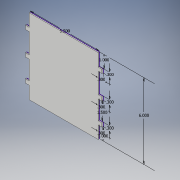
# Autodesk Inventor part: BB Gun Back Panel
Saved by Autodesk Inventor 2018 (Build 220112000, 112)
## iProperties
Created: 2019-05-24
Part Number: BB Gun Back Panel
Material: Generic
Document SubType Name: Modeling
Designer: 871357
Density: 1 g/cm^3
Appearance: Default
Author: 871357
Autodesk Inventor part; units mm, degrees
ref_plane "YZ Plane" through (0, 0, 0) normal (1, 0, 0) x (0, 1, 0)
ref_plane "XZ Plane" through (0, 0, 0) normal (0, 1, 0) x (-1, 0, 0)
ref_plane "XY Plane" through (0, 0, 0) normal (0, 0, 1) x (1, 0, 0)
sketch "Sketch1" plane through (0, 0, 0) normal (0, 0, 1) x (1, 0, 0)
  line L0 (0, 0) -> (139.7, 0)
  line L1 (139.7, 0) -> (139.7, 152.4)
  line L2 (139.7, 152.4) -> (0, 152.4)
  line L3 (139.7, 127) -> (147.32, 127)
  line L4 (147.32, 127) -> (147.32, 119.38)
  line L5 (147.32, 119.38) -> (139.7, 119.38)
  line L6 (139.7, 119.38) -> (139.7, 127)
  line L7 (139.7, 78.74) -> (147.32, 78.74)
  line L8 (147.32, 78.74) -> (147.32, 71.12)
  line L9 (147.32, 71.12) -> (139.7, 71.12)
  line L10 (139.7, 71.12) -> (139.7, 78.74)
  line L11 (139.7, 33.02) -> (147.32, 33.02)
  line L12 (147.32, 33.02) -> (147.32, 25.4)
  line L13 (147.32, 25.4) -> (139.7, 25.4)
  line L14 (139.7, 25.4) -> (139.7, 33.02)
  line L15 (69.85, 152.4) -> (69.85, 0) construction
  line L16 (0, 127) -> (-7.62, 127)
  line L17 (-7.62, 127) -> (-7.62, 119.38)
  line L18 (-7.62, 119.38) -> (0, 119.38)
  line L19 (0, 78.74) -> (-7.62, 78.74)
  line L20 (-7.62, 78.74) -> (-7.62, 71.12)
  line L21 (-7.62, 71.12) -> (0, 71.12)
  line L22 (0, 33.02) -> (-7.62, 33.02)
  line L23 (-7.62, 33.02) -> (-7.62, 25.4)
  line L24 (-7.62, 25.4) -> (0, 25.4)
  line L25 (0, 152.4) -> (0, 127)
  line L26 (0, 119.38) -> (0, 78.74)
  line L27 (0, 71.12) -> (0, 33.02)
  line L28 (0, 25.4) -> (0, 0)
  dimension "d0" = 139.7
  dimension "d1" = 152.4
  dimension "d2" = 7.62
  dimension "d3" = 7.62
  dimension "d4" = 25.4
  dimension "d5" = 7.62
  dimension "d6" = 7.62
  dimension "d7" = 7.62
  dimension "d8" = 7.62
  dimension "d9" = 25.4
  dimension "d10" = 38.1
  constraints: 58 end point, 12 symmetric about line, 11 parallel, 4 horizontal, 4 perpendicular, 3 point on line, 2 midpoint
  measures "d0" distance of L2.end L1.end
  measures "d1" distance of L0.end L1.end
  measures "d2" distance of L4.end L5.end
  measures "d3" distance of L3.end L4.end
  measures "d4" distance between parallel lines of L2 L3
  measures "d5" distance of L8.end L9.end
  measures "d6" distance of L7.end L8.end
  measures "d7" distance of L12.end L13.end
  measures "d8" distance of L11.end L12.end
  measures "d9" distance between parallel lines of L0 L13
  measures "d10" distance between parallel lines of L9 L11
extrude "Extrusion1" add sketch "Sketch1" along normal blind 2.54
body "Solid1"
